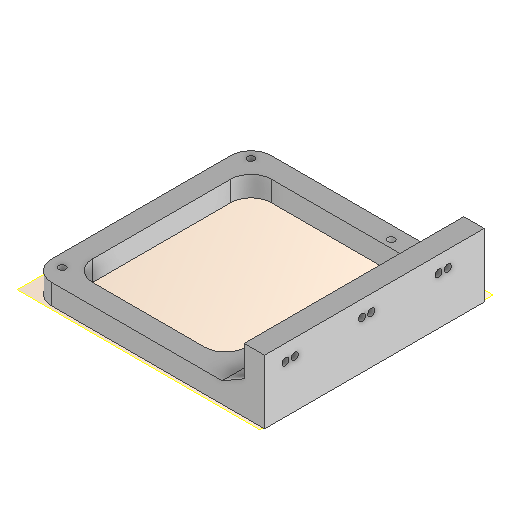
# Autodesk Inventor part: 60_Planktoscope_Electronicsholder
Saved by Autodesk Inventor 2024.1 (Build 281209000, 209)
## iProperties
Created: 2024-07-24
Part Number: 60_Planktoscope_Electronicsholder
Material: Generisch
Document SubType Name: Modeling
Designer: diederichbenedict
Density: 1 g/cm^3
Appearance: Vorgabe
Author: diederichbenedict
Autodesk Inventor part; units mm, degrees
ref_plane "YZ Plane" through (0, 0, 0) normal (1, 0, 0) x (0, 1, 0)
ref_plane "XZ Plane" through (0, 0, 0) normal (0, 1, 0) x (-1, 0, 0)
ref_plane "XY Plane" through (0, 0, 0) normal (0, 0, 1) x (1, 0, 0)
ref_plane "Arbeitsebene1" through (0, 0, 3) normal (0, 0, 1) x (1, 0, 0)
sketch "Skizze1" plane through (0, 0, 3) normal (0, 0, 1) x (1, 0, 0)
  line L0 (43.1941, -41.5994) -> (-43.1659, -41.5994) construction
  line L1 (43.1941, 41.5856) -> (43.1941, -41.5994) construction
  line L2 (-43.2224, 41.5856) -> (43.1941, 41.5856) construction
  line L3 (-43.1659, -41.5994) -> (-43.2224, 41.5856) construction
  circle A0 centre (37.6276, -35.8844) radius 0.5 construction
  circle A1 centre (35.0876, -35.8844) radius 0.5 construction
  circle A2 centre (32.5476, -35.8844) radius 0.5 construction
  circle A3 centre (36.8476, -29.7044) radius 0.5 construction
  circle A4 centre (25.8376, -35.8644) radius 0.5 construction
  circle A5 centre (23.2976, -35.8644) radius 0.5 construction
  circle A6 centre (20.7576, -35.8644) radius 0.5 construction
  circle A7 centre (36.8476, -27.1644) radius 0.5 construction
  circle A8 centre (36.8476, -24.6244) radius 0.5 construction
  circle A9 centre (29.7776, -28.4144) radius 1.6 construction
  circle A10 centre (36.8976, -19.8144) radius 0.5 construction
  circle A11 centre (29.8161, -22.9044) radius 0.5 construction
  circle A12 centre (27.2761, -22.9044) radius 0.5 construction
  circle A13 centre (24.7361, -22.9044) radius 0.5 construction
  circle A14 centre (22.1961, -22.9044) radius 0.5 construction
  circle A15 centre (19.6561, -22.9044) radius 0.5 construction
  circle A16 centre (13.8076, -35.7944) radius 0.5 construction
  circle A17 centre (11.2676, -35.7944) radius 0.5 construction
  circle A18 centre (8.7276, -35.7944) radius 0.5 construction
  circle A19 centre (1.7376, -35.7544) radius 0.5 construction
  circle A20 centre (-0.8024, -35.7544) radius 0.5 construction
  circle A21 centre (18.2361, -29.1444) radius 0.5 construction
  circle A22 centre (18.2361, -26.6044) radius 0.5 construction
  circle A23 centre (10.7361, -29.1444) radius 0.5 construction
  circle A24 centre (10.7361, -26.6044) radius 0.5 construction
  circle A25 centre (17.1161, -22.9044) radius 0.5 construction
  circle A26 centre (14.5761, -22.9044) radius 0.5 construction
  circle A27 centre (12.0361, -22.9044) radius 0.5 construction
  circle A28 centre (9.4961, -22.9044) radius 0.5 construction
  circle A29 centre (3.2361, -29.1444) radius 0.5 construction
  circle A30 centre (3.2361, -26.6044) radius 0.5 construction
  circle A31 centre (6.9561, -22.9044) radius 0.5 construction
  circle A32 centre (1.1961, -20.0044) radius 0.5 construction
  circle A33 centre (36.8976, -17.2744) radius 0.5 construction
  circle A34 centre (36.8976, -14.7344) radius 0.5 construction
  circle A35 centre (36.9476, -8.9644) radius 0.5 construction
  circle A36 centre (36.9476, -6.4244) radius 0.5 construction
  circle A37 centre (30.7111, -6.3544) radius 0.5 construction
  circle A38 centre (36.9476, -3.8844) radius 0.5 construction
  circle A39 centre (30.7111, -3.8144) radius 0.5 construction
  circle A40 centre (30.7111, -1.2744) radius 0.5 construction
  circle A41 centre (5.3111, -6.3544) radius 0.5 construction
  circle A42 centre (5.3111, -3.8144) radius 0.5 construction
  circle A43 centre (5.3111, -1.2744) radius 0.5 construction
  circle A44 centre (-3.3424, -35.7544) radius 0.5 construction
  circle A45 centre (-8.1789, -38.8044) radius 0.5 construction
  circle A46 centre (-8.1789, -35.1044) radius 0.5 construction
  circle A47 centre (-8.1789, -31.4044) radius 0.5 construction
  circle A48 centre (-10.7189, -38.8044) radius 0.5 construction
  circle A49 centre (-10.7189, -35.1044) radius 0.5 construction
  circle A50 centre (-14.5659, -33.6344) radius 0.5 construction
  circle A51 centre (-10.7189, -31.4044) radius 0.5 construction
  circle A52 centre (-17.1059, -33.6344) radius 0.5 construction
  circle A53 centre (-19.6459, -33.6344) radius 0.5 construction
  circle A54 centre (-1.3439, -27.2044) radius 0.5 construction
  circle A55 centre (-3.8839, -27.2044) radius 0.5 construction
  circle A56 centre (-6.4239, -27.2044) radius 0.5 construction
  circle A57 centre (-8.9639, -27.2044) radius 0.5 construction
  circle A58 centre (-1.3439, -23.6044) radius 0.5 construction
  circle A59 centre (-3.8839, -23.6044) radius 0.5 construction
  circle A60 centre (-1.3439, -20.0044) radius 0.5 construction
  circle A61 centre (-3.8839, -20.0044) radius 0.5 construction
  circle A62 centre (-6.4239, -23.6044) radius 0.5 construction
  circle A63 centre (-8.9639, -23.6044) radius 0.5 construction
  circle A64 centre (-6.4239, -20.0044) radius 0.5 construction
  circle A65 centre (-8.9639, -20.0044) radius 0.5 construction
  circle A66 centre (-14.5659, -20.9344) radius 0.5 construction
  circle A67 centre (-17.1059, -20.9344) radius 0.5 construction
  circle A68 centre (-19.6459, -20.9344) radius 0.5 construction
  circle A69 centre (-22.1859, -33.6344) radius 0.5 construction
  circle A70 centre (-24.7259, -33.6344) radius 0.5 construction
  circle A71 centre (-27.2659, -33.6344) radius 0.5 construction
  circle A72 centre (-29.8059, -33.6344) radius 0.5 construction
  circle A73 centre (-38.2224, -37.4144) radius 1.6 construction
  circle A74 centre (-32.3459, -33.6344) radius 0.5 construction
  circle A75 centre (-38.3399, -30.1694) radius 0.5 construction
  circle A76 centre (-22.1859, -20.9344) radius 0.5 construction
  circle A77 centre (-24.7259, -20.9344) radius 0.5 construction
  circle A78 centre (-27.2659, -20.9344) radius 0.5 construction
  circle A79 centre (-29.8059, -20.9344) radius 0.5 construction
  circle A80 centre (-38.3399, -27.6294) radius 0.5 construction
  circle A81 centre (-38.3399, -25.0894) radius 0.5 construction
  circle A82 centre (-32.3459, -20.9344) radius 0.5 construction
  circle A83 centre (-38.3399, -22.5494) radius 0.5 construction
  circle A84 centre (-2.2639, -15.2044) radius 0.375 construction
  circle A85 centre (-4.2639, -15.2044) radius 0.375 construction
  circle A86 centre (-6.2639, -15.2044) radius 0.375 construction
  circle A87 centre (-8.2639, -15.2044) radius 0.375 construction
  circle A88 centre (-2.2639, -9.7044) radius 0.375 construction
  circle A89 centre (-4.2639, -9.7044) radius 0.375 construction
  circle A90 centre (-6.2639, -9.7044) radius 0.375 construction
  circle A91 centre (-8.2639, -9.7044) radius 0.375 construction
  circle A92 centre (-14.5659, -15.6344) radius 0.5 construction
  circle A93 centre (-17.1059, -15.6344) radius 0.5 construction
  circle A94 centre (-19.6459, -15.6344) radius 0.5 construction
  circle A95 centre (-2.2639, -4.2044) radius 0.375 construction
  circle A96 centre (-4.2639, -4.2044) radius 0.375 construction
  circle A97 centre (-6.2639, -4.2044) radius 0.375 construction
  circle A98 centre (-8.2639, -4.2044) radius 0.375 construction
  circle A99 centre (-14.5659, -2.9344) radius 0.5 construction
  circle A100 centre (-17.1059, -2.9344) radius 0.5 construction
  circle A101 centre (-19.6459, -2.9344) radius 0.5 construction
  circle A102 centre (-22.1859, -15.6344) radius 0.5 construction
  circle A103 centre (-24.7259, -15.6344) radius 0.5 construction
  circle A104 centre (-27.2659, -15.6344) radius 0.5 construction
  circle A105 centre (-29.8059, -15.6344) radius 0.5 construction
  circle A106 centre (-32.3459, -15.6344) radius 0.5 construction
  circle A107 centre (-38.4669, -13.2784) radius 0.5 construction
  circle A108 centre (-38.4669, -10.7384) radius 0.5 construction
  circle A109 centre (-22.1859, -2.9344) radius 0.5 construction
  circle A110 centre (-24.7259, -2.9344) radius 0.5 construction
  circle A111 centre (-27.2659, -2.9344) radius 0.5 construction
  circle A112 centre (-29.8059, -2.9344) radius 0.5 construction
  circle A113 centre (-38.4669, -8.1984) radius 0.5 construction
  circle A114 centre (-38.4669, -5.6584) radius 0.5 construction
  circle A115 centre (-32.3459, -2.9344) radius 0.5 construction
  circle A116 centre (36.9476, 0.6556) radius 0.5 construction
  circle A117 centre (36.9476, 3.1956) radius 0.5 construction
  circle A118 centre (30.7111, 1.2656) radius 0.5 construction
  circle A119 centre (30.7111, 3.8056) radius 0.5 construction
  circle A120 centre (36.9476, 5.7356) radius 0.5 construction
  circle A121 centre (30.7111, 6.3456) radius 0.5 construction
  circle A122 centre (30.7111, 8.8856) radius 0.5 construction
  circle A123 centre (36.9976, 10.7656) radius 0.5 construction
  circle A124 centre (36.9976, 13.3056) radius 0.5 construction
  circle A125 centre (30.7111, 11.4256) radius 0.5 construction
  circle A126 centre (30.7111, 13.9656) radius 0.5 construction
  circle A127 centre (36.9976, 15.8456) radius 0.5 construction
  circle A128 centre (30.7111, 16.5056) radius 0.5 construction
  circle A129 centre (30.7111, 19.0456) radius 0.5 construction
  circle A130 centre (5.3111, 1.2656) radius 0.5 construction
  circle A131 centre (5.3111, 3.8056) radius 0.5 construction
  circle A132 centre (5.3111, 6.3456) radius 0.5 construction
  circle A133 centre (5.3111, 8.8856) radius 0.5 construction
  circle A134 centre (5.3111, 11.4256) radius 0.5 construction
  circle A135 centre (5.3111, 13.9656) radius 0.5 construction
  circle A136 centre (5.3111, 16.5056) radius 0.5 construction
  circle A137 centre (5.3111, 19.0456) radius 0.5 construction
  circle A138 centre (36.9476, 20.9456) radius 0.5 construction
  circle A139 centre (36.9476, 23.4856) radius 0.5 construction
  circle A140 centre (30.7111, 21.5856) radius 0.5 construction
  circle A141 centre (30.7111, 24.1256) radius 0.5 construction
  circle A142 centre (36.9476, 26.0256) radius 0.5 construction
  circle A143 centre (30.7111, 26.6656) radius 0.5 construction
  circle A144 centre (30.7111, 29.2056) radius 0.5 construction
  circle A145 centre (30.7111, 31.7456) radius 0.5 construction
  circle A146 centre (30.7111, 34.2856) radius 0.5 construction
  circle A147 centre (30.7111, 36.8256) radius 0.5 construction
  circle A148 centre (30.7111, 39.3656) radius 0.5 construction
  circle A149 centre (5.3111, 21.5856) radius 0.5 construction
  circle A150 centre (5.3111, 24.1256) radius 0.5 construction
  circle A151 centre (5.3111, 26.6656) radius 0.5 construction
  circle A152 centre (5.3111, 29.2056) radius 0.5 construction
  circle A153 centre (16.7776, 36.5856) radius 1.6 construction
  circle A154 centre (5.3111, 31.7456) radius 0.5 construction
  circle A155 centre (5.3111, 34.2856) radius 0.5 construction
  circle A156 centre (5.3111, 36.8256) radius 0.5 construction
  circle A157 centre (5.3111, 39.3656) radius 0.5 construction
  circle A158 centre (-14.5659, 2.3656) radius 0.5 construction
  circle A159 centre (-17.1059, 2.3656) radius 0.5 construction
  circle A160 centre (-19.6459, 2.3656) radius 0.5 construction
  circle A161 centre (-14.5659, 15.0656) radius 0.5 construction
  circle A162 centre (-17.1059, 15.0656) radius 0.5 construction
  circle A163 centre (-19.6459, 15.0656) radius 0.5 construction
  circle A164 centre (-14.5659, 20.0656) radius 0.5 construction
  circle A165 centre (-17.1059, 20.0656) radius 0.5 construction
  circle A166 centre (-19.6459, 20.0656) radius 0.5 construction
  circle A167 centre (-22.1859, 2.3656) radius 0.5 construction
  circle A168 centre (-24.7259, 2.3656) radius 0.5 construction
  circle A169 centre (-27.2659, 2.3656) radius 0.5 construction
  circle A170 centre (-29.8059, 2.3656) radius 0.5 construction
  circle A171 centre (-32.3459, 2.3656) radius 0.5 construction
  circle A172 centre (-38.4669, 4.8826) radius 0.5 construction
  circle A173 centre (-38.4669, 7.4226) radius 0.5 construction
  circle A174 centre (-38.4669, 9.9626) radius 0.5 construction
  circle A175 centre (-22.1859, 15.0656) radius 0.5 construction
  circle A176 centre (-24.7259, 15.0656) radius 0.5 construction
  circle A177 centre (-27.2659, 15.0656) radius 0.5 construction
  circle A178 centre (-29.8059, 15.0656) radius 0.5 construction
  circle A179 centre (-22.1859, 20.0656) radius 0.5 construction
  circle A180 centre (-24.7259, 20.0656) radius 0.5 construction
  circle A181 centre (-27.2659, 20.0656) radius 0.5 construction
  circle A182 centre (-29.8059, 20.0656) radius 0.5 construction
  circle A183 centre (-32.3459, 15.0656) radius 0.5 construction
  circle A184 centre (-38.4669, 12.5026) radius 0.5 construction
  circle A185 centre (-32.3459, 20.0656) radius 0.5 construction
  line L4 (-0.223, 29.8753) -> (-0.0936, 29.8162) construction
  line L5 (-0.0936, 29.8162) -> (0.014, 29.723) construction
  line L6 (0.014, 29.723) -> (0.0909, 29.6033) construction
  line L7 (0.0909, 29.6033) -> (0.131, 29.4667) construction
  line L8 (0.131, 29.4667) -> (0.131, 29.3244) construction
  line L9 (0.131, 29.3244) -> (0.0909, 29.1879) construction
  line L10 (0.0909, 29.1879) -> (0.014, 29.0681) construction
  line L11 (0.014, 29.0681) -> (-0.0936, 28.9749) construction
  line L12 (-0.0936, 28.9749) -> (-0.223, 28.9158) construction
  line L13 (-0.223, 28.9158) -> (-0.3639, 28.8956) construction
  line L14 (-0.3639, 28.8956) -> (-2.9639, 28.8956) construction
  line L15 (-2.9639, 28.8956) -> (-3.1047, 28.9158) construction
  line L16 (-3.1047, 28.9158) -> (-3.2342, 28.9749) construction
  line L17 (-3.2342, 28.9749) -> (-3.3417, 29.0681) construction
  line L18 (-3.3417, 29.0681) -> (-3.4187, 29.1879) construction
  line L19 (-3.4187, 29.1879) -> (-3.4588, 29.3244) construction
  line L20 (-3.4588, 29.3244) -> (-3.4588, 29.4667) construction
  line L21 (-3.4588, 29.4667) -> (-3.4187, 29.6033) construction
  line L22 (-3.4187, 29.6033) -> (-3.3417, 29.723) construction
  line L23 (-3.3417, 29.723) -> (-3.2342, 29.8162) construction
  line L24 (-3.2342, 29.8162) -> (-3.1047, 29.8753) construction
  line L25 (-3.1047, 29.8753) -> (-2.9639, 29.8956) construction
  line L26 (-2.9639, 29.8956) -> (-0.3639, 29.8956) construction
  line L27 (-0.3639, 29.8956) -> (-0.223, 29.8753) construction
  line L28 (-6.9436, 33.5364) -> (-6.8845, 33.6659) construction
  line L29 (-6.8845, 33.6659) -> (-6.7913, 33.7734) construction
  line L30 (-6.7913, 33.7734) -> (-6.6716, 33.8504) construction
  line L31 (-6.6716, 33.8504) -> (-6.535, 33.8905) construction
  line L32 (-6.535, 33.8905) -> (-6.3927, 33.8905) construction
  line L33 (-6.3927, 33.8905) -> (-6.2562, 33.8504) construction
  line L34 (-6.2562, 33.8504) -> (-6.1364, 33.7734) construction
  line L35 (-6.1364, 33.7734) -> (-6.0432, 33.6659) construction
  line L36 (-6.0432, 33.6659) -> (-5.9841, 33.5364) construction
  line L37 (-5.9841, 33.5364) -> (-5.9639, 33.3956) construction
  line L38 (-5.9639, 33.3956) -> (-5.9639, 31.1956) construction
  line L39 (-5.9639, 31.1956) -> (-5.9841, 31.0547) construction
  line L40 (-5.9841, 31.0547) -> (-6.0432, 30.9253) construction
  line L41 (-6.0432, 30.9253) -> (-6.1364, 30.8177) construction
  line L42 (-6.1364, 30.8177) -> (-6.2562, 30.7408) construction
  line L43 (-6.2562, 30.7408) -> (-6.3927, 30.7007) construction
  line L44 (-6.3927, 30.7007) -> (-6.535, 30.7007) construction
  line L45 (-6.535, 30.7007) -> (-6.6716, 30.7408) construction
  line L46 (-6.6716, 30.7408) -> (-6.7913, 30.8177) construction
  line L47 (-6.7913, 30.8177) -> (-6.8845, 30.9253) construction
  line L48 (-6.8845, 30.9253) -> (-6.9436, 31.0547) construction
  line L49 (-6.9436, 31.0547) -> (-6.9639, 31.1956) construction
  line L50 (-6.9639, 31.1956) -> (-6.9639, 33.3956) construction
  line L51 (-6.9639, 33.3956) -> (-6.9436, 33.5364) construction
  line L52 (-0.423, 36.1753) -> (-0.2936, 36.1162) construction
  line L53 (-0.2936, 36.1162) -> (-0.186, 36.023) construction
  line L54 (-0.186, 36.023) -> (-0.1091, 35.9033) construction
  line L55 (-0.1091, 35.9033) -> (-0.069, 35.7667) construction
  line L56 (-0.069, 35.7667) -> (-0.069, 35.6244) construction
  line L57 (-0.069, 35.6244) -> (-0.1091, 35.4879) construction
  line L58 (-0.1091, 35.4879) -> (-0.186, 35.3681) construction
  line L59 (-0.186, 35.3681) -> (-0.2936, 35.2749) construction
  line L60 (-0.2936, 35.2749) -> (-0.423, 35.2158) construction
  line L61 (-0.423, 35.2158) -> (-0.5639, 35.1956) construction
  line L62 (-0.5639, 35.1956) -> (-2.7639, 35.1956) construction
  line L63 (-2.7639, 35.1956) -> (-2.9047, 35.2158) construction
  line L64 (-2.9047, 35.2158) -> (-3.0342, 35.2749) construction
  line L65 (-3.0342, 35.2749) -> (-3.1417, 35.3681) construction
  line L66 (-3.1417, 35.3681) -> (-3.2187, 35.4879) construction
  line L67 (-3.2187, 35.4879) -> (-3.2588, 35.6244) construction
  line L68 (-3.2588, 35.6244) -> (-3.2588, 35.7667) construction
  line L69 (-3.2588, 35.7667) -> (-3.2187, 35.9033) construction
  line L70 (-3.2187, 35.9033) -> (-3.1417, 36.023) construction
  line L71 (-3.1417, 36.023) -> (-3.0342, 36.1162) construction
  line L72 (-3.0342, 36.1162) -> (-2.9047, 36.1753) construction
  line L73 (-2.9047, 36.1753) -> (-2.7639, 36.1956) construction
  line L74 (-2.7639, 36.1956) -> (-0.5639, 36.1956) construction
  line L75 (-0.5639, 36.1956) -> (-0.423, 36.1753) construction
  circle A186 centre (-14.5659, 32.7656) radius 0.5 construction
  circle A187 centre (-17.1059, 32.7656) radius 0.5 construction
  circle A188 centre (-19.6459, 32.7656) radius 0.5 construction
  circle A189 centre (-38.4669, 22.1546) radius 0.5 construction
  circle A190 centre (-38.4669, 24.6946) radius 0.5 construction
  circle A191 centre (-38.4669, 27.2346) radius 0.5 construction
  circle A192 centre (-38.4669, 29.7746) radius 0.5 construction
  circle A193 centre (-22.1859, 32.7656) radius 0.5 construction
  circle A194 centre (-24.7259, 32.7656) radius 0.5 construction
  circle A195 centre (-27.2659, 32.7656) radius 0.5 construction
  circle A196 centre (-29.8059, 32.7656) radius 0.5 construction
  circle A197 centre (-32.3459, 32.7656) radius 0.5 construction
  circle A198 centre (-38.2224, 36.5856) radius 1.6 construction
  line L76 (48.1941, 113.9931) -> (48.1941, -93.0069) projected
  line L77 (-43.2224, 41.5856) -> (48.1941, 41.5856)
  line L78 (48.1941, 41.5856) -> (48.1941, -44.5117)
  line L79 (48.1941, -44.5117) -> (-43.2224, -44.5117)
  line L80 (-43.2224, -44.5117) -> (-43.2224, 41.5856)
  line L81 (-35.2224, -36.5117) -> (40.1941, -36.5117)
  line L82 (40.1941, -36.5117) -> (40.1941, 33.5856)
  line L83 (40.1941, 33.5856) -> (-35.2224, 33.5856)
  line L84 (-35.2224, 33.5856) -> (-35.2224, -36.5117)
  line L85 (24.7361, -36.5117) -> (40.1941, -36.5117)
  line L86 (40.1941, -36.5117) -> (40.1941, -23.4063)
  line L87 (40.1941, -23.4063) -> (24.7361, -23.4063)
  line L88 (24.7361, -23.4063) -> (24.7361, -36.5117)
  circle A199 centre (-38.2224, -37.4144) radius 1.4
  circle A200 centre (29.7776, -28.4144) radius 1.4
  circle A201 centre (16.7776, 36.5856) radius 1.4
  circle A202 centre (-38.2224, 36.5856) radius 1.4
  point P0 (0, 0)
  point P1 (48.1941, 41.5856)
  dimension "d0" = 8
  dimension "d1" = 2.8
  dimension "d2" = 2.8
  dimension "d3" = 2.8
  dimension "d4" = 2.8
  constraints: 24 end point, 6 parallel, 4 centre point, 4 coincident, 3 perpendicular, 3 point on line, 2 horizontal, 3 other
  measures "d0" distance between parallel lines of L79 L81
  measures "d1" diameter of A199
  measures "d2" diameter of A200
  measures "d3" diameter of A201
  measures "d4" diameter of A202
extrude "Extrusion1" add sketch "Skizze1" along normal blind 8 contours L76 L79 L80 L77 | L88 L87 L82 L81
sketch "Skizze2" plane through (48.1941, -44.5117, 3) normal (1, 0, 0) x (0, 0, -1)
  line L0 (0, 86.0973) -> (-8, 86.0973) projected
  line L1 (0, 0) -> (-8, 0) projected
  line L2 (-41.7258, 75.9615) -> (-41.7258, 34.048) projected
  line L3 (-41.7258, 34.048) -> (-71.8357, 34.048) projected
  line L4 (-71.8357, 34.048) -> (-71.8357, 75.9615) projected
  line L5 (-71.8357, 75.9615) -> (-41.7258, 75.9615) projected
  circle A0 centre (-54.852, -47.3333) radius 1.4 projected
  circle A1 centre (-39.852, -47.3333) radius 1.4 projected
  circle A2 centre (-18.7192, 8.1964) radius 1.4 projected
  circle A3 centre (-18.7192, 38.1964) radius 1.4 projected
  circle A4 centre (-18.7192, 68.1964) radius 1.4 projected
  circle A5 centre (-18.7192, 98.1964) radius 1.4 projected
  circle A6 centre (-18.7192, 128.1964) radius 1.4 projected
  circle A7 centre (-69.852, -47.3333) radius 1.4 projected
  circle A8 centre (-69.852, 157.3428) radius 1.4 projected
  circle A9 centre (-54.852, 157.3428) radius 1.4 projected
  circle A10 centre (-39.852, 157.3428) radius 1.4 projected
  circle A11 centre (-18.7192, 101.8131) radius 1.4 projected
  circle A12 centre (-18.7192, 71.8131) radius 1.4 projected
  circle A13 centre (-18.7192, 41.8131) radius 1.4 projected
  circle A14 centre (-18.7192, 11.8131) radius 1.4 projected
  circle A15 centre (-18.7192, -18.1869) radius 1.4 projected
  circle A16 centre (-115.652, 158.5048) radius 1.4 projected
  circle A17 centre (33.348, 158.5048) radius 1.4 projected
  circle A18 centre (33.348, -48.4952) radius 1.4 projected
  circle A19 centre (-115.652, -48.4952) radius 1.4 projected
  circle A20 centre (-33.552, -2.4952) radius 1.5746 projected
  circle A21 centre (-48.3, -2.4952) radius 1.5746 projected
  circle A22 centre (-32, 113.5048) radius 1.5746 projected
  circle A23 centre (-49.852, 113.5048) radius 1.5746 projected
  circle A24 centre (-76.152, -2.4952) radius 1.5746 projected
  circle A25 centre (-61.4039, -2.4952) radius 1.5746 projected
  circle A26 centre (-77.7039, 113.5048) radius 1.5746 projected
  circle A27 centre (-59.852, 113.5048) radius 1.5746 projected
  line L6 (-115.652, 173.3302) -> (33.348, 173.3302) projected
  arc A28 (-115.652, 173.3302) -> (-130.4774, 158.5048) centre (-115.652, 158.5048) ccw projected
  line L7 (-130.4774, -48.4952) -> (-130.4774, 158.5048) projected
  arc A29 (-130.4774, -48.4952) -> (-115.652, -63.3207) centre (-115.652, -48.4952) ccw projected
  line L8 (33.348, -63.3207) -> (-115.652, -63.3207) projected
  arc A30 (33.348, -63.3207) -> (48.1735, -48.4952) centre (33.348, -48.4952) ccw projected
  line L9 (48.1735, -40.6698) -> (48.1735, -48.4952) projected
  line L10 (41.848, -40.6698) -> (48.1735, -40.6698) projected
  arc A31 (26.6735, -25.4952) -> (41.848, -40.6698) centre (41.848, -25.4952) ccw projected
  line L11 (26.6735, -16.0952) -> (26.6735, -25.4952) projected
  arc A32 (41.848, -0.9207) -> (26.6735, -16.0952) centre (41.848, -16.0952) ccw projected
  line L12 (48.1735, -0.9207) -> (41.848, -0.9207) projected
  line L13 (48.1735, 158.5048) -> (48.1735, -0.9207) projected
  arc A33 (48.1735, 158.5048) -> (33.348, 173.3302) centre (33.348, 158.5048) ccw projected
  line L14 (-8, 0) -> (-8, 86.0973) projected
  line L15 (-8, 86.0973) -> (-25, 86.0973)
  line L16 (-25, 86.0973) -> (-25, 0)
  line L17 (-25, 0) -> (-8, 0)
  line L18 (-8, 0) -> (-8, 86.0973)
  line L19 (-91.152, -21.4995) -> (8.848, -21.4995) projected
  arc A34 (8.848, -41.4995) -> (8.848, -21.4995) centre (8.848, -31.4995) ccw projected
  line L20 (8.848, -41.4995) -> (-91.152, -41.4995) projected
  arc A35 (-91.152, -21.4995) -> (-91.152, -41.4995) centre (-91.152, -31.4995) ccw projected
  line L21 (-91.152, 150.8178) -> (8.848, 150.8178) projected
  arc A36 (8.848, 130.8178) -> (8.848, 150.8178) centre (8.848, 140.8178) ccw projected
  line L22 (8.848, 130.8178) -> (-91.152, 130.8178) projected
  arc A37 (-91.152, 150.8178) -> (-91.152, 130.8178) centre (-91.152, 140.8178) ccw projected
  point P0 (3, 44.5117)
  dimension "d7" = 17
  constraints: 8 end point, 2 parallel, 1 horizontal, 1 perpendicular
  measures "d7" distance of L17.end L16.end
extrude "Extrusion2" add sketch "Skizze2" against normal up to surface (8 mm away) contours L17 L16 L15 L14
chamfer "Fasen1" distance 5 angle 60 2 edges at (40.1941, 37.5856, 11) (40.1941, -33.959, 11) measured on face at (40.1941, -33.959, 11.5) measured on face at (40.1941, 37.5856, 11.5)
fillet "Rundung1" radius 8 8 edges at (-43.2224, 41.5856, 7) (-43.2224, -44.5117, 7) (-35.2224, -36.5117, 7) (-35.2224, 33.5856, 7) (24.7361, -36.5117, 7) (24.7361, -23.4063, 7) (40.1941, -23.4063, 13.5) (40.1941, -23.4063, 7)
